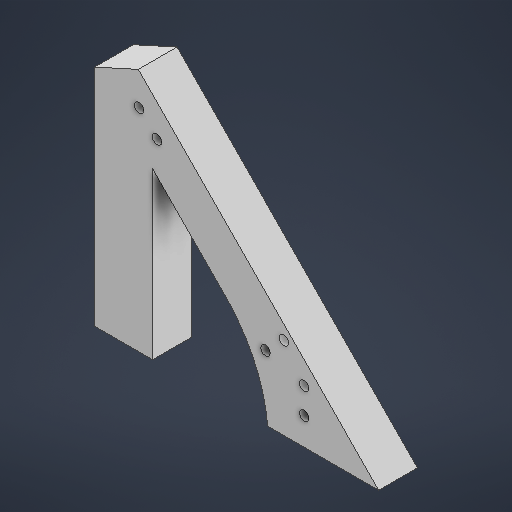
# Autodesk Inventor part: Lady Brown Brace
Saved by Autodesk Inventor 2025 (Build 290162000, 162)
## iProperties
Created: 2024-12-19
Part Number: Lady Brown Brace
Material: Generic
Document SubType Name: Modeling
Designer: Juan
Density: 1 g/cm^3
Appearance: Default
Author: Juan
Autodesk Inventor part; units mm, degrees
ref_plane "YZ Plane" through (0, 0, 0) normal (1, 0, 0) x (0, 1, 0)
ref_plane "XZ Plane" through (0, 0, 0) normal (0, 1, 0) x (-1, 0, 0)
ref_plane "XY Plane" through (0, 0, 0) normal (0, 0, 1) x (1, 0, 0)
sketch "Sketch1" plane through (0, 0, 0) normal (0, 0, 1) x (1, 0, 0)
  line L0 (-28.8758, -59.7214) -> (-28.8758, 21.7165)
  line L1 (-18.8555, -59.7214) -> (-80.3235, -59.7214)
  line L2 (-57.4508, -59.7214) -> (-57.4508, 50.7628)
  line L3 (-28.8758, 21.7165) -> (27.7449, -35.838)
  line L4 (27.7449, -35.838) -> (27.7449, -59.7214)
  line L5 (-57.4508, 50.7628) -> (-35.9111, 60.559)
  line L6 (-35.9111, 60.559) -> (82.4177, -59.7214)
  line L7 (82.4177, -59.7214) -> (27.7449, -59.7214)
  arc A0 (27.7449, -59.7214) -> (8.6214, -16.3991) centre (-46.0524, -66.4154) ccw
  circle A1 centre (45.7367, -33.5276) radius 2.3241
  circle A2 centre (45.7367, -46.2276) radius 2.3241
  circle A3 centre (26.6867, -27.9714) radius 2.3241
  circle A4 centre (35.7401, -19.0649) radius 2.3241
  circle A5 centre (-35.5854, 44.3824) radius 2.3241
  circle A6 centre (-26.6789, 35.329) radius 2.3241
  point P0 (0, 0)
  dimension "d0" = 90
  dimension "d1" = 90
  dimension "d2" = 4.6482
  dimension "d3" = 4.6482
  dimension "d4" = 4.6482
  dimension "d5" = 4.6482
  dimension "d6" = 4.6482
  dimension "d7" = 4.6482
  constraints: 16 end point, 7 centre point, 2 point on circle, 2 point on line, 1 vertical
  measures "d0" angle of L2 L1
  measures "d1" angle of L7 L4
  measures "d2" diameter of A1
  measures "d3" diameter of A2
  measures "d4" diameter of A3
  measures "d5" diameter of A4
  measures "d6" diameter of A5
  measures "d7" diameter of A6
extrude "Extrusion1" add sketch "Sketch1" along normal blind 19.0627
sketch "Sketch2" plane through (0, 0, 0) normal (0, 0, -1) x (-1, 0, 0)
  line L0 (28.8758, -59.7214) -> (28.8758, 21.7165) projected
  line L1 (57.4508, -59.7214) -> (28.8758, -59.7214) projected
  line L2 (57.4508, 50.7628) -> (57.4508, -59.7214) projected
  line L3 (28.8758, -59.7214) -> (30.4633, -59.7214)
  line L4 (57.4508, -59.7214) -> (55.8633, -59.7214)
  line L5 (30.4633, -59.7214) -> (30.4633, -46.2594)
  line L6 (30.4633, -46.2594) -> (55.8633, -46.2594)
  line L7 (55.8633, -46.2594) -> (55.8633, -59.7214)
  line L8 (28.8758, -59.7214) -> (28.8758, -46.2594)
  line L9 (30.4633, -46.2594) -> (28.8758, -46.2594)
  line L10 (55.8633, -46.2594) -> (57.4508, -46.2594)
  line L11 (57.4508, -59.7214) -> (57.4508, -46.2594)
  point P0 (0, 0)
  dimension "d10" = 1.5875
  dimension "d11" = 1.5875
  dimension "d12" = 13.462
  constraints: 18 end point, 5 point on line, 3 perpendicular, 1 collinear, 1 vertical
  measures "d10" distance of L0.start L3.end
  measures "d11" distance of L1.start L4.end
  measures "d12" distance of L3.end L5.end
extrude "Extrusion2" cut sketch "Sketch2" against normal blind 17.4752 contours L5 L6 L7 L1
body "Solid1"
